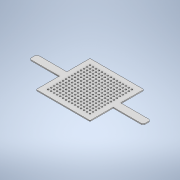
# Autodesk Inventor part: MouldCover20x20
Saved by Autodesk Inventor 2020.3 (Build 243373010, 373A)
## iProperties
Created: 2020-10-26
Part Number: MouldCover20x20
Material: Generic
Document SubType Name: Modeling
Designer: Naude Conradie
Density: 1 g/cm^3
Appearance: Default
Author: Naude Conradie
Autodesk Inventor part; units mm, degrees
ref_plane "YZ Plane" through (0, 0, 0) normal (1, 0, 0) x (0, 1, 0)
ref_plane "XZ Plane" through (0, 0, 0) normal (0, 1, 0) x (-1, 0, 0)
ref_plane "XY Plane" through (0, 0, 0) normal (0, 0, 1) x (1, 0, 0)
sketch "Sketch1" plane through (0, 0, 0) normal (0, 1, 0) x (-1, 0, 0)
  line L0 (0, 0) -> (180, 0)
  line L1 (180, 0) -> (180, -180)
  line L2 (180, -180) -> (0, -180)
  line L3 (0, -180) -> (0, 0)
  dimension "d0" = 180
  dimension "d1" = 180
  constraints: 8 end point, 2 parallel, 1 horizontal, 1 perpendicular
  measures "d0" distance of L1.end L2.end
  measures "d1" distance of L0.end L1.end
extrude "Extrusion1" add sketch "Sketch1" along normal blind 3
sketch "Sketch2" plane through (0, 3, 0) normal (0, 1, 0) x (1, 0, 0)
  line L0 (-180, 0) -> (0, 0) projected
  line L1 (0, 0) -> (0, 180) projected
  point P0 (-20, 20)
  point P1 (-30, 20)
  point P2 (-40, 20)
  point P3 (-50, 20)
  point P4 (-60, 20)
  point P5 (-70, 20)
  point P6 (-80, 20)
  point P7 (-90, 20)
  point P8 (-100, 20)
  point P9 (-110, 20)
  point P10 (-120, 20)
  point P11 (-130, 20)
  point P12 (-140, 20)
  point P13 (-150, 20)
  point P14 (-160, 20)
  point P15 (-20, 30)
  point P16 (-30, 30)
  point P17 (-40, 30)
  point P18 (-50, 30)
  point P19 (-60, 30)
  point P20 (-70, 30)
  point P21 (-80, 30)
  point P22 (-90, 30)
  point P23 (-100, 30)
  point P24 (-110, 30)
  point P25 (-120, 30)
  point P26 (-130, 30)
  point P27 (-140, 30)
  point P28 (-150, 30)
  point P29 (-160, 30)
  point P30 (-20, 40)
  point P31 (-30, 40)
  point P32 (-40, 40)
  point P33 (-50, 40)
  point P34 (-60, 40)
  point P35 (-70, 40)
  point P36 (-80, 40)
  point P37 (-90, 40)
  point P38 (-100, 40)
  point P39 (-110, 40)
  point P40 (-120, 40)
  point P41 (-130, 40)
  point P42 (-140, 40)
  point P43 (-150, 40)
  point P44 (-160, 40)
  point P45 (-20, 50)
  point P46 (-30, 50)
  point P47 (-40, 50)
  point P48 (-50, 50)
  point P49 (-60, 50)
  point P50 (-70, 50)
  point P51 (-80, 50)
  point P52 (-90, 50)
  point P53 (-100, 50)
  point P54 (-110, 50)
  point P55 (-120, 50)
  point P56 (-130, 50)
  point P57 (-140, 50)
  point P58 (-150, 50)
  point P59 (-160, 50)
  point P60 (-20, 60)
  point P61 (-30, 60)
  point P62 (-40, 60)
  point P63 (-50, 60)
  point P64 (-60, 60)
  point P65 (-70, 60)
  point P66 (-80, 60)
  point P67 (-90, 60)
  point P68 (-100, 60)
  point P69 (-110, 60)
  point P70 (-120, 60)
  point P71 (-130, 60)
  point P72 (-140, 60)
  point P73 (-150, 60)
  point P74 (-160, 60)
  point P75 (-20, 70)
  point P76 (-30, 70)
  point P77 (-40, 70)
  point P78 (-50, 70)
  point P79 (-60, 70)
  point P80 (-70, 70)
  point P81 (-80, 70)
  point P82 (-90, 70)
  point P83 (-100, 70)
  point P84 (-110, 70)
  point P85 (-120, 70)
  point P86 (-130, 70)
  point P87 (-140, 70)
  point P88 (-150, 70)
  point P89 (-160, 70)
  point P90 (-20, 80)
  point P91 (-30, 80)
  point P92 (-40, 80)
  point P93 (-50, 80)
  point P94 (-60, 80)
  point P95 (-70, 80)
  point P96 (-80, 80)
  point P97 (-90, 80)
  point P98 (-100, 80)
  point P99 (-110, 80)
  point P100 (-120, 80)
  point P101 (-130, 80)
  point P102 (-140, 80)
  point P103 (-150, 80)
  point P104 (-160, 80)
  point P105 (-20, 90)
  point P106 (-30, 90)
  point P107 (-40, 90)
  point P108 (-50, 90)
  point P109 (-60, 90)
  point P110 (-70, 90)
  point P111 (-80, 90)
  point P112 (-90, 90)
  point P113 (-100, 90)
  point P114 (-110, 90)
  point P115 (-120, 90)
  point P116 (-130, 90)
  point P117 (-140, 90)
  point P118 (-150, 90)
  point P119 (-160, 90)
  point P120 (-20, 100)
  point P121 (-30, 100)
  point P122 (-40, 100)
  point P123 (-50, 100)
  point P124 (-60, 100)
  point P125 (-70, 100)
  point P126 (-80, 100)
  point P127 (-90, 100)
  point P128 (-100, 100)
  point P129 (-110, 100)
  point P130 (-120, 100)
  point P131 (-130, 100)
  point P132 (-140, 100)
  point P133 (-150, 100)
  point P134 (-160, 100)
  point P135 (-20, 110)
  point P136 (-30, 110)
  point P137 (-40, 110)
  point P138 (-50, 110)
  point P139 (-60, 110)
  point P140 (-70, 110)
  point P141 (-80, 110)
  point P142 (-90, 110)
  point P143 (-100, 110)
  point P144 (-110, 110)
  point P145 (-120, 110)
  point P146 (-130, 110)
  point P147 (-140, 110)
  point P148 (-150, 110)
  point P149 (-160, 110)
  point P150 (-20, 120)
  point P151 (-30, 120)
  point P152 (-40, 120)
  point P153 (-50, 120)
  point P154 (-60, 120)
  point P155 (-70, 120)
  point P156 (-80, 120)
  point P157 (-90, 120)
  point P158 (-100, 120)
  point P159 (-110, 120)
  point P160 (-120, 120)
  point P161 (-130, 120)
  point P162 (-140, 120)
  point P163 (-150, 120)
  point P164 (-160, 120)
  point P165 (-20, 130)
  point P166 (-30, 130)
  point P167 (-40, 130)
  point P168 (-50, 130)
  point P169 (-60, 130)
  point P170 (-70, 130)
  point P171 (-80, 130)
  point P172 (-90, 130)
  point P173 (-100, 130)
  point P174 (-110, 130)
  point P175 (-120, 130)
  point P176 (-130, 130)
  point P177 (-140, 130)
  point P178 (-150, 130)
  point P179 (-160, 130)
  point P180 (-20, 140)
  point P181 (-30, 140)
  point P182 (-40, 140)
  point P183 (-50, 140)
  point P184 (-60, 140)
  point P185 (-70, 140)
  point P186 (-80, 140)
  point P187 (-90, 140)
  point P188 (-100, 140)
  point P189 (-110, 140)
  point P190 (-120, 140)
  point P191 (-130, 140)
  point P192 (-140, 140)
  point P193 (-150, 140)
  point P194 (-160, 140)
  point P195 (-20, 150)
  point P196 (-30, 150)
  point P197 (-40, 150)
  point P198 (-50, 150)
  point P199 (-60, 150)
  dimension "d4" = 20
  dimension "d5" = 20
  dimension "d8" = 10
  dimension "d11" = 10
  constraints: 1 horizontal, 1 vertical, 224 other
  measures "d4" distance from line of L0 point (-20, 20)
  measures "d5" distance from line of L1 point (-20, 20)
  measures "d8" distance of point (-20, 20) point (-30, 20)
  measures "d11" distance of point (-20, 20) point (-20, 30)
hole "Hole1" at (-20, 3, -20) at (-30, 3, -20) at (-40, 3, -20) at (-50, 3, -20) at (-60, 3, -20) at (-70, 3, -20) at (-80, 3, -20) at (-90, 3, -20) at (-100, 3, -20) at (-110, 3, -20) at (-120, 3, -20) at (-130, 3, -20) at (-140, 3, -20) at (-150, 3, -20) at (-160, 3, -20) at (-20, 3, -30) at (-30, 3, -30) at (-40, 3, -30) at (-50, 3, -30) at (-60, 3, -30) at (-70, 3, -30) at (-80, 3, -30) at (-90, 3, -30) at (-100, 3, -30) at (-110, 3, -30) at (-120, 3, -30) at (-130, 3, -30) at (-140, 3, -30) at (-150, 3, -30) at (-160, 3, -30) at (-20, 3, -40) at (-30, 3, -40) at (-40, 3, -40) at (-50, 3, -40) at (-60, 3, -40) at (-70, 3, -40) at (-80, 3, -40) at (-90, 3, -40) at (-100, 3, -40) at (-110, 3, -40) at (-120, 3, -40) at (-130, 3, -40) at (-140, 3, -40) at (-150, 3, -40) at (-160, 3, -40) at (-20, 3, -50) at (-30, 3, -50) at (-40, 3, -50) at (-50, 3, -50) at (-60, 3, -50) direction (0, -1, 0) diameter 5 end through all and at (-70, 3, -50) (-80, 3, -50) (-90, 3, -50) (-100, 3, -50) (-110, 3, -50) (-120, 3, -50) (-130, 3, -50) (-140, 3, -50) (-150, 3, -50) (-160, 3, -50) (-20, 3, -60) (-30, 3, -60) (-40, 3, -60) (-50, 3, -60) (-60, 3, -60) (-70, 3, -60) (-80, 3, -60) (-90, 3, -60) (-100, 3, -60) (-110, 3, -60) (-120, 3, -60) (-130, 3, -60) (-140, 3, -60) (-150, 3, -60) (-160, 3, -60) (-20, 3, -70) (-30, 3, -70) (-40, 3, -70) (-50, 3, -70) (-60, 3, -70) (-70, 3, -70) (-80, 3, -70) (-90, 3, -70) (-100, 3, -70) (-110, 3, -70) (-120, 3, -70) (-130, 3, -70) (-140, 3, -70) (-150, 3, -70) (-160, 3, -70) (-20, 3, -80) (-30, 3, -80) (-40, 3, -80) (-50, 3, -80) (-60, 3, -80) (-70, 3, -80) (-80, 3, -80) (-90, 3, -80) (-100, 3, -80) (-110, 3, -80) (-120, 3, -80) (-130, 3, -80) (-140, 3, -80) (-150, 3, -80) (-160, 3, -80) (-20, 3, -90) (-30, 3, -90) (-40, 3, -90) (-50, 3, -90) (-60, 3, -90) (-70, 3, -90) (-80, 3, -90) (-90, 3, -90) (-100, 3, -90) (-110, 3, -90) (-120, 3, -90) (-130, 3, -90) (-140, 3, -90) (-150, 3, -90) (-160, 3, -90) (-20, 3, -100) (-30, 3, -100) (-40, 3, -100) (-50, 3, -100) (-60, 3, -100) (-70, 3, -100) (-80, 3, -100) (-90, 3, -100) (-100, 3, -100) (-110, 3, -100) (-120, 3, -100) (-130, 3, -100) (-140, 3, -100) (-150, 3, -100) (-160, 3, -100) (-20, 3, -110) (-30, 3, -110) (-40, 3, -110) (-50, 3, -110) (-60, 3, -110) (-70, 3, -110) (-80, 3, -110) (-90, 3, -110) (-100, 3, -110) (-110, 3, -110) (-120, 3, -110) (-130, 3, -110) (-140, 3, -110) (-150, 3, -110) (-160, 3, -110) (-20, 3, -120) (-30, 3, -120) (-40, 3, -120) (-50, 3, -120) (-60, 3, -120) (-70, 3, -120) (-80, 3, -120) (-90, 3, -120) (-100, 3, -120) (-110, 3, -120) (-120, 3, -120) (-130, 3, -120) (-140, 3, -120) (-150, 3, -120) (-160, 3, -120) (-20, 3, -130) (-30, 3, -130) (-40, 3, -130) (-50, 3, -130) (-60, 3, -130) (-70, 3, -130) (-80, 3, -130) (-90, 3, -130) (-100, 3, -130) (-110, 3, -130) (-120, 3, -130) (-130, 3, -130) (-140, 3, -130) (-150, 3, -130) (-160, 3, -130) (-20, 3, -140) (-30, 3, -140) (-40, 3, -140) (-50, 3, -140) (-60, 3, -140) (-70, 3, -140) (-80, 3, -140) (-90, 3, -140) (-100, 3, -140) (-110, 3, -140) (-120, 3, -140) (-130, 3, -140) (-140, 3, -140) (-150, 3, -140) (-160, 3, -140) (-20, 3, -150) (-30, 3, -150) (-40, 3, -150) (-50, 3, -150) (-60, 3, -150) (-70, 3, -150) (-80, 3, -150) (-90, 3, -150) (-100, 3, -150) (-110, 3, -150) (-120, 3, -150) (-130, 3, -150) (-140, 3, -150) (-150, 3, -150) (-160, 3, -150) (-20, 3, -160) (-30, 3, -160) (-40, 3, -160) (-50, 3, -160) (-60, 3, -160) (-70, 3, -160) (-80, 3, -160) (-90, 3, -160) (-100, 3, -160) (-110, 3, -160) (-120, 3, -160) (-130, 3, -160) (-140, 3, -160) (-150, 3, -160) (-160, 3, -160)
chamfer "Chamfer1" distance 2 angle 45 4 edges at (-180, 1.5, -180) (0, 1.5, -180) (0, 1.5, 0) (-180, 1.5, 0)
sketch "Sketch3" plane through (0, 0, -2) normal (1, 0, 0) x (0, 0, -1)
  line L0 (0, 3) -> (176, 3) projected
  line L1 (176, 3) -> (0, 3) projected
  line L2 (75.5, 0) -> (100.5, 0)
  line L3 (100.5, 0) -> (100.5, 3)
  line L4 (100.5, 3) -> (75.5, 3)
  line L5 (75.5, 3) -> (75.5, 0)
  point P0 (-2, 0)
  point P1 (75.5, 3)
  dimension "d24" = 25
  dimension "d25" = 77.5
  constraints: 8 end point, 2 parallel, 1 horizontal, 1 perpendicular, 1 point on line
  measures "d24" distance of L4.end L3.end
  measures "d25" distance of L2.start point (-2, 0)
extrude "Extrusion2" add sketch "Sketch3" along normal blind 100
sketch "Sketch4" plane through (-180, 0, -178) normal (-1, 0, 0) x (0, 0, 1)
  line L0 (0, 3) -> (176, 3) projected
  line L1 (70.5, 0) -> (65.5, 0) projected
  line L2 (75.5, 0) -> (100.5, 0)
  line L3 (100.5, 0) -> (100.5, 3)
  line L4 (100.5, 3) -> (75.5, 3)
  line L5 (75.5, 3) -> (75.5, 0)
  line L6 (-2, 3) -> (-2, 0) projected
  point P0 (178, 0)
  dimension "d28" = 25
  dimension "d29" = 77.5
  constraints: 8 end point, 2 parallel, 2 point on line, 1 horizontal, 1 perpendicular
  measures "d28" distance of L4.end L3.end
  measures "d29" distance from line of L6 L2.start
extrude "Extrusion3" add sketch "Sketch4" along normal blind 100
chamfer "Chamfer2" distance 5 angle 45 4 edges at (-280, 1.5, -77.5) (-280, 1.5, -102.5) (100, 1.5, -102.5) (100, 1.5, -77.5)
body "Solid1"
